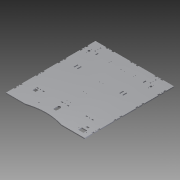
# Autodesk Inventor part: Esquena
Saved by Autodesk Inventor 2012 SP1 (Build 160190100, 190)
## iProperties
Created: 2015-01-06
Part Number: Esquena
Material: Default
Document SubType Name: Modeling
Designer: PRINCIPAL
Density: 1 g/cm^3
Author: PRINCIPAL
Autodesk Inventor part; units mm, degrees
ref_plane "YZ Plane" through (0, 0, 0) normal (1, 0, 0) x (0, 1, 0)
ref_plane "XZ Plane" through (0, 0, 0) normal (0, 1, 0) x (-1, 0, 0)
ref_plane "XY Plane" through (0, 0, 0) normal (0, 0, 1) x (1, 0, 0)
sketch "Boceto1" plane through (0, 0, 0) normal (0, 0, 1) x (1, 0, 0)
  line L0 (-140.4962, 506.797) -> (-140.4962, 516.797)
  arc A0 (-135.4962, 516.797) -> (-140.4962, 516.797) centre (-137.9962, 516.797) ccw
  line L1 (-135.4962, 516.797) -> (-135.4962, 506.797)
  arc A1 (-140.4962, 506.797) -> (-135.4962, 506.797) centre (-137.9962, 506.797) ccw
  line L2 (102.8213, 506.797) -> (102.8213, 516.797)
  arc A2 (107.8213, 516.797) -> (102.8213, 516.797) centre (105.3213, 516.797) ccw
  line L3 (107.8213, 516.797) -> (107.8213, 506.797)
  arc A3 (102.8213, 506.797) -> (107.8213, 506.797) centre (105.3213, 506.797) ccw
  line L4 (-142.9962, 204.2587) -> (-127.9962, 204.2587)
  line L5 (-127.9962, 204.2587) -> (-127.9962, 189.2587)
  line L6 (-127.9962, 189.2587) -> (-142.9962, 189.2587)
  line L7 (-142.9962, 189.2587) -> (-142.9962, 204.2587)
  line L8 (-141.3535, 416.9103) -> (-136.3535, 416.9103)
  line L9 (-136.3535, 416.9103) -> (-136.3535, 396.9103)
  line L10 (-136.3535, 396.9103) -> (-141.3535, 396.9103)
  line L11 (-141.3535, 396.9103) -> (-141.3535, 416.9103)
  line L12 (-125.3535, 416.9103) -> (-120.3535, 416.9103)
  line L13 (-120.3535, 416.9103) -> (-120.3535, 396.9103)
  line L14 (-120.3535, 396.9103) -> (-125.3535, 396.9103)
  line L15 (-125.3535, 396.9103) -> (-125.3535, 416.9103)
  line L16 (105.2713, 214.272) -> (115.1713, 214.272)
  line L17 (115.1713, 214.272) -> (115.1713, 209.322)
  line L18 (115.1713, 209.322) -> (105.2713, 209.322)
  line L19 (105.2713, 209.322) -> (105.2713, 214.272)
  line L20 (10.2713, 214.272) -> (20.1713, 214.272)
  line L21 (20.1713, 214.272) -> (20.1713, 209.322)
  line L22 (20.1713, 209.322) -> (10.2713, 209.322)
  line L23 (10.2713, 209.322) -> (10.2713, 214.272)
  line L24 (-19.7287, 214.272) -> (-9.8287, 214.272)
  line L25 (-9.8287, 214.272) -> (-9.8287, 209.322)
  line L26 (-9.8287, 209.322) -> (-19.7287, 209.322)
  line L27 (-19.7287, 209.322) -> (-19.7287, 214.272)
  line L28 (-114.7287, 209.322) -> (-114.7287, 214.272)
  line L29 (-114.7287, 214.272) -> (-104.8287, 214.272)
  line L30 (-104.8287, 214.272) -> (-104.8287, 209.322)
  line L31 (-104.8287, 209.322) -> (-114.7287, 209.322)
  line L32 (135.2713, 214.272) -> (145.1713, 214.272)
  line L33 (145.1713, 214.272) -> (145.1713, 209.322)
  line L34 (145.1713, 209.322) -> (135.2713, 209.322)
  line L35 (135.2713, 209.322) -> (135.2713, 214.272)
  line L36 (-134.8287, 214.272) -> (-134.8287, 209.322)
  line L37 (-134.8287, 209.322) -> (-144.7287, 209.322)
  line L38 (-144.7287, 209.322) -> (-144.7287, 214.272)
  line L39 (-144.7287, 214.272) -> (-134.8287, 214.272)
  line L40 (-153.3037, 519.314) -> (-158.2537, 519.314)
  line L41 (-158.2537, 519.314) -> (-158.2537, 524.2799)
  line L42 (-158.2537, 524.2799) -> (-153.3037, 524.2799)
  line L43 (-153.3037, 524.2799) -> (-153.3037, 519.314)
  line L44 (-158.2537, 550.2799) -> (-153.3037, 550.2799)
  line L45 (-153.3037, 550.2799) -> (-153.3037, 545.314)
  line L46 (-153.3037, 545.314) -> (-158.2537, 545.314)
  line L47 (-158.2537, 545.314) -> (-158.2537, 550.2799)
  line L48 (128.1803, 545.322) -> (123.2303, 545.322)
  line L49 (123.2303, 545.322) -> (123.2303, 550.272)
  line L50 (123.2303, 550.272) -> (128.1803, 550.272)
  line L51 (128.1803, 550.272) -> (128.1803, 545.322)
  line L52 (128.1803, 519.322) -> (123.2303, 519.322)
  line L53 (123.2303, 519.322) -> (123.2303, 524.272)
  line L54 (123.2303, 524.272) -> (128.1803, 524.272)
  line L55 (128.1803, 524.272) -> (128.1803, 519.322)
  line L56 (195.3213, 384.697) -> (200.3213, 384.697)
  line L57 (200.3213, 384.697) -> (200.3213, 404.897)
  line L58 (200.3213, 404.897) -> (195.3213, 404.897)
  line L59 (195.3213, 404.897) -> (195.3213, 414.697)
  line L60 (195.3213, 414.697) -> (200.3213, 414.697)
  line L61 (200.3213, 414.697) -> (200.3213, 486.897)
  line L62 (200.3213, 486.897) -> (195.3213, 486.897)
  line L63 (195.3213, 486.897) -> (195.3213, 496.697)
  line L64 (195.3213, 496.697) -> (200.3213, 496.697)
  line L65 (200.3213, 496.697) -> (200.3213, 516.897)
  line L66 (200.3213, 516.897) -> (195.3213, 516.897)
  line L67 (195.3213, 516.897) -> (195.3213, 526.697)
  line L68 (195.3213, 526.697) -> (200.3213, 526.697)
  line L69 (200.3213, 526.697) -> (200.3213, 566.897)
  line L70 (200.3213, 566.897) -> (145.1213, 566.897)
  line L71 (145.1213, 566.897) -> (145.1213, 561.897)
  line L72 (145.1213, 561.897) -> (135.3213, 561.897)
  line L73 (135.3213, 561.897) -> (135.3213, 566.897)
  line L74 (135.3213, 566.897) -> (115.1213, 566.897)
  line L75 (115.1213, 566.897) -> (115.1213, 561.897)
  line L76 (115.1213, 561.897) -> (105.3213, 561.897)
  line L77 (105.3213, 561.897) -> (105.3213, 566.897)
  line L78 (105.3213, 566.897) -> (20.1213, 566.897)
  line L79 (20.1213, 566.897) -> (20.1213, 561.897)
  line L80 (20.1213, 561.897) -> (10.3213, 561.897)
  line L81 (10.3213, 561.897) -> (10.3213, 566.897)
  line L82 (10.3213, 566.897) -> (-9.8787, 566.897)
  line L83 (-9.8787, 566.897) -> (-9.8787, 561.897)
  line L84 (-9.8787, 561.897) -> (-19.6787, 561.897)
  line L85 (-19.6787, 561.897) -> (-19.6787, 566.897)
  line L86 (-19.6787, 566.897) -> (-104.8656, 566.897)
  line L87 (-104.8656, 566.897) -> (-104.8656, 561.897)
  line L88 (-104.8656, 561.897) -> (-114.6787, 561.897)
  line L89 (-114.6787, 561.897) -> (-114.6787, 566.897)
  line L90 (-114.6787, 566.897) -> (-134.8787, 566.897)
  line L91 (-134.8787, 566.897) -> (-134.8787, 561.897)
  line L92 (-134.8787, 561.897) -> (-144.6787, 561.897)
  line L93 (-144.6787, 561.897) -> (-144.6787, 566.897)
  line L94 (-144.6787, 566.897) -> (-199.8787, 566.897)
  line L95 (-199.8787, 566.897) -> (-199.8787, 526.697)
  line L96 (-199.8787, 526.697) -> (-194.8787, 526.697)
  line L97 (-194.8787, 526.697) -> (-194.8787, 516.897)
  line L98 (-194.8787, 516.897) -> (-199.8787, 516.897)
  line L99 (-199.8787, 516.897) -> (-199.8787, 496.697)
  line L100 (-199.8787, 496.697) -> (-194.8787, 496.697)
  line L101 (-194.8787, 496.697) -> (-194.8787, 486.897)
  line L102 (-194.8787, 486.897) -> (-199.8787, 486.897)
  line L103 (-199.8787, 486.897) -> (-199.8787, 414.697)
  line L104 (-199.8787, 414.697) -> (-194.8787, 414.697)
  line L105 (-194.8787, 414.697) -> (-194.8787, 404.897)
  line L106 (-194.8787, 404.897) -> (-199.8787, 404.897)
  line L107 (-199.8787, 404.897) -> (-199.8787, 384.697)
  line L108 (-199.8787, 384.697) -> (-194.8787, 384.697)
  line L109 (-194.8787, 384.697) -> (-194.8787, 374.897)
  line L110 (-194.8787, 374.897) -> (-199.8787, 374.897)
  line L111 (-199.8787, 374.897) -> (-199.8787, 302.697)
  line L112 (-199.8787, 302.697) -> (-194.8787, 302.697)
  line L113 (-194.8787, 302.697) -> (-194.8787, 292.897)
  line L114 (-194.8787, 292.897) -> (-199.8787, 292.897)
  line L115 (-199.8787, 292.897) -> (-199.8787, 272.697)
  line L116 (-199.8787, 272.697) -> (-194.8787, 272.697)
  line L117 (-194.8787, 272.697) -> (-194.8787, 262.897)
  line L118 (-194.8787, 262.897) -> (-199.8787, 262.897)
  line L119 (-199.8787, 262.897) -> (-199.8787, 190.697)
  line L120 (-199.8787, 190.697) -> (-194.8787, 190.697)
  line L121 (-194.8787, 190.697) -> (-194.8787, 180.897)
  line L122 (-194.8787, 180.897) -> (-199.8787, 180.897)
  line L123 (-199.8787, 180.897) -> (-199.8787, 160.697)
  line L124 (-199.8787, 160.697) -> (-194.8787, 160.697)
  line L125 (-194.8787, 160.697) -> (-194.8787, 150.897)
  line L126 (-194.8787, 150.897) -> (-199.8787, 150.897)
  line L127 (-199.8787, 150.897) -> (-199.8787, 110.697)
  line L128 (-199.8787, 110.697) -> (-102.2877, 110.697)
  arc A4 (-102.2877, 110.697) -> (-87.1428, 114.7846) centre (-128.2484, 236.9821) ccw
  arc A5 (67.462, 114.7846) -> (-87.1428, 114.7846) centre (-9.8404, -158.132) ccw
  arc A6 (67.462, 114.7846) -> (82.6069, 110.697) centre (1623.1793, 5848.6689) ccw
  line L129 (82.6069, 110.697) -> (200.3213, 110.697)
  line L130 (200.3213, 110.697) -> (200.3213, 150.897)
  line L131 (200.3213, 150.897) -> (195.3213, 150.897)
  line L132 (195.3213, 150.897) -> (195.3213, 160.697)
  line L133 (195.3213, 160.697) -> (200.3213, 160.697)
  line L134 (200.3213, 160.697) -> (200.3213, 180.897)
  line L135 (200.3213, 180.897) -> (195.3213, 180.897)
  line L136 (195.3213, 180.897) -> (195.3213, 190.697)
  line L137 (195.3213, 190.697) -> (200.3213, 190.697)
  line L138 (200.3213, 190.697) -> (200.3213, 262.897)
  line L139 (200.3213, 262.897) -> (195.3213, 262.897)
  line L140 (195.3213, 262.897) -> (195.3213, 272.697)
  line L141 (195.3213, 272.697) -> (200.3213, 272.697)
  line L142 (200.3213, 272.697) -> (200.3213, 292.897)
  line L143 (200.3213, 292.897) -> (195.3213, 292.897)
  line L144 (195.3213, 292.897) -> (195.3213, 302.697)
  line L145 (195.3213, 302.697) -> (200.3213, 302.697)
  line L146 (200.3213, 302.697) -> (200.3213, 374.897)
  line L147 (200.3213, 374.897) -> (195.3213, 374.897)
  line L148 (195.3213, 374.897) -> (195.3213, 384.697)
  arc A7 (125.7213, 536.347) -> (124.1713, 534.797) centre (125.7213, 534.797) ccw
  arc A8 (124.1713, 534.797) -> (125.7213, 533.247) centre (125.7213, 534.797) ccw
  arc A9 (125.7213, 533.247) -> (127.2713, 534.797) centre (125.7213, 534.797) ccw
  arc A10 (127.2713, 534.797) -> (125.7213, 536.347) centre (125.7213, 534.797) ccw
  arc A11 (-155.7787, 536.347) -> (-157.3287, 534.797) centre (-155.7787, 534.797) ccw
  arc A12 (-157.3287, 534.797) -> (-155.7787, 533.247) centre (-155.7787, 534.797) ccw
  arc A13 (-155.7787, 533.247) -> (-154.2287, 534.797) centre (-155.7787, 534.797) ccw
  arc A14 (-154.2287, 534.797) -> (-155.7787, 536.347) centre (-155.7787, 534.797) ccw
  arc A15 (142.7213, 495.847) -> (141.1713, 494.297) centre (142.7213, 494.297) ccw
  arc A16 (141.1713, 494.297) -> (142.7213, 492.747) centre (142.7213, 494.297) ccw
  arc A17 (142.7213, 492.747) -> (144.2713, 494.297) centre (142.7213, 494.297) ccw
  arc A18 (144.2713, 494.297) -> (142.7213, 495.847) centre (142.7213, 494.297) ccw
  arc A19 (-172.7787, 495.847) -> (-174.3287, 494.297) centre (-172.7787, 494.297) ccw
  arc A20 (-174.3287, 494.297) -> (-172.7787, 492.747) centre (-172.7787, 494.297) ccw
  arc A21 (-172.7787, 492.747) -> (-171.2287, 494.297) centre (-172.7787, 494.297) ccw
  arc A22 (-171.2287, 494.297) -> (-172.7787, 495.847) centre (-172.7787, 494.297) ccw
  arc A23 (-172.7787, 520.847) -> (-174.3287, 519.297) centre (-172.7787, 519.297) ccw
  arc A24 (-174.3287, 519.297) -> (-172.7787, 517.747) centre (-172.7787, 519.297) ccw
  arc A25 (-172.7787, 517.747) -> (-171.2287, 519.297) centre (-172.7787, 519.297) ccw
  arc A26 (-171.2287, 519.297) -> (-172.7787, 520.847) centre (-172.7787, 519.297) ccw
  arc A27 (142.7213, 520.847) -> (141.1713, 519.297) centre (142.7213, 519.297) ccw
  arc A28 (141.1713, 519.297) -> (142.7213, 517.747) centre (142.7213, 519.297) ccw
  arc A29 (142.7213, 517.747) -> (144.2713, 519.297) centre (142.7213, 519.297) ccw
  arc A30 (144.2713, 519.297) -> (142.7213, 520.847) centre (142.7213, 519.297) ccw
  arc A31 (125.2213, 566.297) -> (123.2213, 564.297) centre (125.2213, 564.297) ccw
  arc A32 (123.2213, 564.297) -> (125.2213, 562.297) centre (125.2213, 564.297) ccw
  arc A33 (125.2213, 562.297) -> (127.2213, 564.297) centre (125.2213, 564.297) ccw
  arc A34 (127.2213, 564.297) -> (125.2213, 566.297) centre (125.2213, 564.297) ccw
  arc A35 (0.2213, 566.297) -> (-1.7787, 564.297) centre (0.2213, 564.297) ccw
  arc A36 (-1.7787, 564.297) -> (0.2213, 562.297) centre (0.2213, 564.297) ccw
  arc A37 (0.2213, 562.297) -> (2.2213, 564.297) centre (0.2213, 564.297) ccw
  arc A38 (2.2213, 564.297) -> (0.2213, 566.297) centre (0.2213, 564.297) ccw
  arc A39 (-124.7787, 566.297) -> (-126.7787, 564.297) centre (-124.7787, 564.297) ccw
  arc A40 (-126.7787, 564.297) -> (-124.7787, 562.297) centre (-124.7787, 564.297) ccw
  arc A41 (-124.7787, 562.297) -> (-122.7787, 564.297) centre (-124.7787, 564.297) ccw
  arc A42 (-122.7787, 564.297) -> (-124.7787, 566.297) centre (-124.7787, 564.297) ccw
  arc A43 (-124.7787, 213.797) -> (-126.7787, 211.797) centre (-124.7787, 211.797) ccw
  arc A44 (-126.7787, 211.797) -> (-124.7787, 209.797) centre (-124.7787, 211.797) ccw
  arc A45 (-124.7787, 209.797) -> (-122.7787, 211.797) centre (-124.7787, 211.797) ccw
  arc A46 (-122.7787, 211.797) -> (-124.7787, 213.797) centre (-124.7787, 211.797) ccw
  arc A47 (-197.2787, 172.797) -> (-199.2787, 170.797) centre (-197.2787, 170.797) ccw
  arc A48 (-199.2787, 170.797) -> (-197.2787, 168.797) centre (-197.2787, 170.797) ccw
  arc A49 (-197.2787, 168.797) -> (-195.2787, 170.797) centre (-197.2787, 170.797) ccw
  arc A50 (-195.2787, 170.797) -> (-197.2787, 172.797) centre (-197.2787, 170.797) ccw
  arc A51 (-197.2787, 396.797) -> (-199.2787, 394.797) centre (-197.2787, 394.797) ccw
  arc A52 (-199.2787, 394.797) -> (-197.2787, 392.797) centre (-197.2787, 394.797) ccw
  arc A53 (-197.2787, 392.797) -> (-195.2787, 394.797) centre (-197.2787, 394.797) ccw
  arc A54 (-195.2787, 394.797) -> (-197.2787, 396.797) centre (-197.2787, 394.797) ccw
  arc A55 (197.7213, 172.797) -> (195.7213, 170.797) centre (197.7213, 170.797) ccw
  arc A56 (195.7213, 170.797) -> (197.7213, 168.797) centre (197.7213, 170.797) ccw
  arc A57 (197.7213, 168.797) -> (199.7213, 170.797) centre (197.7213, 170.797) ccw
  arc A58 (199.7213, 170.797) -> (197.7213, 172.797) centre (197.7213, 170.797) ccw
  arc A59 (197.7213, 396.797) -> (195.7213, 394.797) centre (197.7213, 394.797) ccw
  arc A60 (195.7213, 394.797) -> (197.7213, 392.797) centre (197.7213, 394.797) ccw
  arc A61 (197.7213, 392.797) -> (199.7213, 394.797) centre (197.7213, 394.797) ccw
  arc A62 (199.7213, 394.797) -> (197.7213, 396.797) centre (197.7213, 394.797) ccw
  arc A63 (197.7213, 508.797) -> (195.7213, 506.797) centre (197.7213, 506.797) ccw
  arc A64 (195.7213, 506.797) -> (197.7213, 504.797) centre (197.7213, 506.797) ccw
  arc A65 (197.7213, 504.797) -> (199.7213, 506.797) centre (197.7213, 506.797) ccw
  arc A66 (199.7213, 506.797) -> (197.7213, 508.797) centre (197.7213, 506.797) ccw
  arc A67 (197.7213, 284.797) -> (195.7213, 282.797) centre (197.7213, 282.797) ccw
  arc A68 (195.7213, 282.797) -> (197.7213, 280.797) centre (197.7213, 282.797) ccw
  arc A69 (197.7213, 280.797) -> (199.7213, 282.797) centre (197.7213, 282.797) ccw
  arc A70 (199.7213, 282.797) -> (197.7213, 284.797) centre (197.7213, 282.797) ccw
  arc A71 (-197.2787, 508.797) -> (-199.2787, 506.797) centre (-197.2787, 506.797) ccw
  arc A72 (-199.2787, 506.797) -> (-197.2787, 504.797) centre (-197.2787, 506.797) ccw
  arc A73 (-197.2787, 504.797) -> (-195.2787, 506.797) centre (-197.2787, 506.797) ccw
  arc A74 (-195.2787, 506.797) -> (-197.2787, 508.797) centre (-197.2787, 506.797) ccw
  arc A75 (125.2213, 213.797) -> (123.2213, 211.797) centre (125.2213, 211.797) ccw
  arc A76 (123.2213, 211.797) -> (125.2213, 209.797) centre (125.2213, 211.797) ccw
  arc A77 (125.2213, 209.797) -> (127.2213, 211.797) centre (125.2213, 211.797) ccw
  arc A78 (127.2213, 211.797) -> (125.2213, 213.797) centre (125.2213, 211.797) ccw
  arc A79 (0.2213, 213.797) -> (-1.7787, 211.797) centre (0.2213, 211.797) ccw
  arc A80 (-1.7787, 211.797) -> (0.2213, 209.797) centre (0.2213, 211.797) ccw
  arc A81 (0.2213, 209.797) -> (2.2213, 211.797) centre (0.2213, 211.797) ccw
  arc A82 (2.2213, 211.797) -> (0.2213, 213.797) centre (0.2213, 211.797) ccw
  arc A83 (-197.2787, 284.797) -> (-199.2787, 282.797) centre (-197.2787, 282.797) ccw
  arc A84 (-199.2787, 282.797) -> (-197.2787, 280.797) centre (-197.2787, 282.797) ccw
  arc A85 (-197.2787, 280.797) -> (-195.2787, 282.797) centre (-197.2787, 282.797) ccw
  arc A86 (-195.2787, 282.797) -> (-197.2787, 284.797) centre (-197.2787, 282.797) ccw
  arc A87 (142.7213, 511.997) -> (137.5213, 506.797) centre (142.7213, 506.797) ccw
  arc A88 (137.5213, 506.797) -> (142.7213, 501.597) centre (142.7213, 506.797) ccw
  arc A89 (142.7213, 501.597) -> (147.9213, 506.797) centre (142.7213, 506.797) ccw
  arc A90 (147.9213, 506.797) -> (142.7213, 511.997) centre (142.7213, 506.797) ccw
  arc A91 (-172.7787, 512.012) -> (-177.9937, 506.797) centre (-172.7787, 506.797) ccw
  arc A92 (-177.9937, 506.797) -> (-172.7787, 501.582) centre (-172.7787, 506.797) ccw
  arc A93 (-172.7787, 501.582) -> (-167.5637, 506.797) centre (-172.7787, 506.797) ccw
  arc A94 (-167.5637, 506.797) -> (-172.7787, 512.012) centre (-172.7787, 506.797) ccw
  arc A95 (-7.7787, 398.297) -> (-9.2787, 396.797) centre (-7.7787, 396.797) ccw
  arc A96 (-9.2787, 396.797) -> (-7.7787, 395.297) centre (-7.7787, 396.797) ccw
  arc A97 (-7.7787, 395.297) -> (-6.2787, 396.797) centre (-7.7787, 396.797) ccw
  arc A98 (-6.2787, 396.797) -> (-7.7787, 398.297) centre (-7.7787, 396.797) ccw
  arc A99 (-70.1004, 518.297) -> (-71.6004, 516.797) centre (-70.1004, 516.797) ccw
  arc A100 (-71.6004, 516.797) -> (-70.1004, 515.297) centre (-70.1004, 516.797) ccw
  arc A101 (-70.1004, 515.297) -> (-68.6004, 516.797) centre (-70.1004, 516.797) ccw
  arc A102 (-68.6004, 516.797) -> (-70.1004, 518.297) centre (-70.1004, 516.797) ccw
  arc A103 (-70.1004, 508.297) -> (-71.6004, 506.797) centre (-70.1004, 506.797) ccw
  arc A104 (-71.6004, 506.797) -> (-70.1004, 505.297) centre (-70.1004, 506.797) ccw
  arc A105 (-70.1004, 505.297) -> (-68.6004, 506.797) centre (-70.1004, 506.797) ccw
  arc A106 (-68.6004, 506.797) -> (-70.1004, 508.297) centre (-70.1004, 506.797) ccw
  arc A107 (53.5107, 518.297) -> (52.0107, 516.797) centre (53.5107, 516.797) ccw
  arc A108 (52.0107, 516.797) -> (53.5107, 515.297) centre (53.5107, 516.797) ccw
  arc A109 (53.5107, 515.297) -> (55.0107, 516.797) centre (53.5107, 516.797) ccw
  arc A110 (55.0107, 516.797) -> (53.5107, 518.297) centre (53.5107, 516.797) ccw
  arc A111 (53.5107, 508.297) -> (52.0107, 506.797) centre (53.5107, 506.797) ccw
  arc A112 (52.0107, 506.797) -> (53.5107, 505.297) centre (53.5107, 506.797) ccw
  arc A113 (53.5107, 505.297) -> (55.0107, 506.797) centre (53.5107, 506.797) ccw
  arc A114 (55.0107, 506.797) -> (53.5107, 508.297) centre (53.5107, 506.797) ccw
  arc A115 (-7.7787, 231.5765) -> (-9.2787, 230.0765) centre (-7.7787, 230.0765) ccw
  arc A116 (-9.2787, 230.0765) -> (-7.7787, 228.5765) centre (-7.7787, 230.0765) ccw
  arc A117 (-7.7787, 228.5765) -> (-6.2787, 230.0765) centre (-7.7787, 230.0765) ccw
  arc A118 (-6.2787, 230.0765) -> (-7.7787, 231.5765) centre (-7.7787, 230.0765) ccw
  arc A119 (8.2213, 231.5765) -> (6.7213, 230.0765) centre (8.2213, 230.0765) ccw
  arc A120 (6.7213, 230.0765) -> (8.2213, 228.5765) centre (8.2213, 230.0765) ccw
  arc A121 (8.2213, 228.5765) -> (9.7213, 230.0765) centre (8.2213, 230.0765) ccw
  arc A122 (9.7213, 230.0765) -> (8.2213, 231.5765) centre (8.2213, 230.0765) ccw
  arc A123 (8.2213, 398.297) -> (6.7213, 396.797) centre (8.2213, 396.797) ccw
  arc A124 (6.7213, 396.797) -> (8.2213, 395.297) centre (8.2213, 396.797) ccw
  arc A125 (8.2213, 395.297) -> (9.7213, 396.797) centre (8.2213, 396.797) ccw
  arc A126 (9.7213, 396.797) -> (8.2213, 398.297) centre (8.2213, 396.797) ccw
  arc A127 (-7.7787, 506.797) -> (-9.2787, 505.297) centre (-7.7787, 505.297) ccw
  arc A128 (-9.2787, 505.297) -> (-7.7787, 503.797) centre (-7.7787, 505.297) ccw
  arc A129 (-7.7787, 503.797) -> (-6.2787, 505.297) centre (-7.7787, 505.297) ccw
  arc A130 (-6.2787, 505.297) -> (-7.7787, 506.797) centre (-7.7787, 505.297) ccw
  arc A131 (8.2213, 506.797) -> (6.7213, 505.297) centre (8.2213, 505.297) ccw
  arc A132 (6.7213, 505.297) -> (8.2213, 503.797) centre (8.2213, 505.297) ccw
  arc A133 (8.2213, 503.797) -> (9.7213, 505.297) centre (8.2213, 505.297) ccw
  arc A134 (9.7213, 505.297) -> (8.2213, 506.797) centre (8.2213, 505.297) ccw
  arc A135 (-71.8787, 152.947) -> (-74.1287, 150.697) centre (-71.8787, 150.697) ccw
  arc A136 (-74.1287, 150.697) -> (-71.8787, 148.447) centre (-71.8787, 150.697) ccw
  arc A137 (-71.8787, 148.447) -> (-69.6287, 150.697) centre (-71.8787, 150.697) ccw
  arc A138 (-69.6287, 150.697) -> (-71.8787, 152.947) centre (-71.8787, 150.697) ccw
  arc A139 (-8, 165.589) -> (0, 157.589) centre (0, 165.589) ccw
  arc A140 (0, 157.589) -> (8, 165.589) centre (0, 165.589) ccw
  line L149 (8, 165.589) -> (8, 180.897)
  arc A141 (8, 180.897) -> (-8, 180.897) centre (0, 180.897) ccw
  line L150 (-8, 180.897) -> (-8, 165.589)
  arc A142 (-7.7787, 315.4556) -> (-9.2787, 313.9556) centre (-7.7787, 313.9556) ccw
  arc A143 (-9.2787, 313.9556) -> (-7.7787, 312.4556) centre (-7.7787, 313.9556) ccw
  arc A144 (-7.7787, 312.4556) -> (-6.2787, 313.9556) centre (-7.7787, 313.9556) ccw
  arc A145 (-6.2787, 313.9556) -> (-7.7787, 315.4556) centre (-7.7787, 313.9556) ccw
  arc A146 (8.2213, 315.4556) -> (6.7213, 313.9556) centre (8.2213, 313.9556) ccw
  arc A147 (6.7213, 313.9556) -> (8.2213, 312.4556) centre (8.2213, 313.9556) ccw
  arc A148 (8.2213, 312.4556) -> (9.7213, 313.9556) centre (8.2213, 313.9556) ccw
  arc A149 (9.7213, 313.9556) -> (8.2213, 315.4556) centre (8.2213, 313.9556) ccw
  line L151 (154.2289, 161.0776) -> (167.6289, 161.0776)
  line L152 (167.6289, 161.0776) -> (167.6289, 169.2776)
  line L153 (167.6289, 169.2776) -> (154.2289, 169.2776)
  line L154 (154.2289, 169.2776) -> (154.2289, 161.0776)
  line L155 (147.4579, 148.188) -> (147.4579, 132.788)
  arc A150 (147.4579, 132.788) -> (149.5579, 130.688) centre (149.5579, 132.788) ccw
  line L156 (149.5579, 130.688) -> (172.8579, 130.688)
  arc A151 (172.8579, 130.688) -> (174.9579, 132.788) centre (172.8579, 132.788) ccw
  line L157 (174.9579, 132.788) -> (174.9579, 148.188)
  arc A152 (174.9579, 148.188) -> (172.8579, 150.288) centre (172.8579, 148.188) ccw
  line L158 (172.8579, 150.288) -> (149.5579, 150.288)
  arc A153 (149.5579, 150.288) -> (147.4579, 148.188) centre (149.5579, 148.188) ccw
  arc A154 (141.2052, 142.238) -> (139.4552, 140.488) centre (141.2052, 140.488) ccw
  arc A155 (139.4552, 140.488) -> (141.2052, 138.738) centre (141.2052, 140.488) ccw
  arc A156 (141.2052, 138.738) -> (142.9552, 140.488) centre (141.2052, 140.488) ccw
  arc A157 (142.9552, 140.488) -> (141.2052, 142.238) centre (141.2052, 140.488) ccw
  arc A158 (181.2013, 142.238) -> (179.4513, 140.488) centre (181.2013, 140.488) ccw
  arc A159 (179.4513, 140.488) -> (181.2013, 138.738) centre (181.2013, 140.488) ccw
  arc A160 (181.2013, 138.738) -> (182.9513, 140.488) centre (181.2013, 140.488) ccw
  arc A161 (182.9513, 140.488) -> (181.2013, 142.238) centre (181.2013, 140.488) ccw
  line L159 (90.8913, 416.9103) -> (95.8913, 416.9103)
  line L160 (95.8913, 416.9103) -> (95.8913, 396.9103)
  line L161 (95.8913, 396.9103) -> (90.8913, 396.9103)
  line L162 (90.8913, 396.9103) -> (90.8913, 416.9103)
  line L163 (106.8913, 416.9103) -> (111.8913, 416.9103)
  line L164 (111.8913, 416.9103) -> (111.8913, 396.9103)
  line L165 (111.8913, 396.9103) -> (106.8913, 396.9103)
  line L166 (106.8913, 396.9103) -> (106.8913, 416.9103)
  point P0 (0, 0)
  constraints: 334 end point, 324 point on circle, 162 centre point
extrude "Extrusión2" add sketch "Boceto1" along normal blind 5
